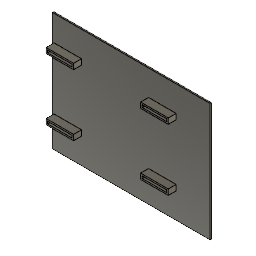
etage v3 (Autodesk Fusion 360 design; units mm, degrees)
Autodesk Fusion 360 part; units mm, degrees
sketch "Sketch1" plane through (0, 0, 0) normal (0, 1, 0) x (1, 0, 0)
  line L0 (0, 0) -> (200, 0)
  line L1 (200, 0) -> (200, -150)
  line L2 (200, -150) -> (0, -150)
  line L3 (0, -150) -> (0, 0)
  dimension "d1" = 200
  dimension "d2" = 150
extrude "Extrude1" add sketch "Sketch1" along normal blind 2
sketch "Sketch2" plane through (0, 0, 0) normal (0, -1, 0) x (1, 0, 0)
  line L0 (200, 150) -> (0, 150)
  line L1 (0, 150) -> (0, 0)
  line L2 (0, 0) -> (200, 0)
  line L3 (200, 0) -> (200, 150)
  line L4 (4, 112.5) -> (35, 112.5)
  line L5 (35, 112.5) -> (35, 115.5)
  line L6 (35, 115.5) -> (4, 115.5)
  line L7 (4, 115.5) -> (4, 112.5)
  line L8 (37, 117.5) -> (2, 117.5)
  line L9 (2, 117.5) -> (2, 110.5)
  line L10 (2, 110.5) -> (37, 110.5)
  line L11 (37, 110.5) -> (37, 117.5)
  line L12 (200, 150) -> (0, 150)
  line L13 (0, 150) -> (0, 0)
  line L14 (0, 0) -> (200, 0)
  line L15 (200, 0) -> (200, 150)
  line L16 (2, 110.5) -> (37, 110.5)
  line L17 (200, 150) -> (0, 150)
  line L18 (0, 150) -> (0, 0)
  line L19 (0, 150) -> (0, 0)
  line L20 (35, 37.5) -> (35, 34.5)
  line L21 (0, 0) -> (200, 0)
  line L22 (122, 39.5) -> (157, 39.5)
  line L23 (35, 112.5) -> (35, 115.5)
  line L24 (37, 110.5) -> (2, 110.5)
  line L25 (2, 110.5) -> (2, 117.5)
  line L26 (2, 117.5) -> (37, 117.5)
  line L27 (37, 117.5) -> (37, 110.5)
  dimension "d5" = 31
  dimension "d6" = 3
  dimension "d7" = 35
  dimension "d8" = 7
  dimension "d9" = 2
  dimension "d10" = 2
  dimension "d18" = 32.5
  dimension "d19" = 2
  measures "d5" distance of L1.end
  measures "d7" distance of L1.end
  measures "d9" distance of L6 L8
  measures "d10" distance of L5 L11
  measures "d17" distance of L16
  measures "d18" distance of L8 L17
  measures "d19" distance of L9 L18
  measures "d37" distance of L22
extrude "Extrude2" add sketch "Sketch2" along normal blind 10 contours L8 L9 L10 L11 L16 L24 L25 L26 L27
sketch "Sketch3" plane through (0, 0, 0) normal (0, -1, 0) x (1, 0, 0)
  line L0 (200, 150) -> (0, 150)
  line L1 (0, 150) -> (0, 0)
  line L2 (0, 0) -> (200, 0)
  line L3 (200, 0) -> (200, 150)
  line L4 (4, 37.5) -> (35, 37.5)
  line L5 (35, 37.5) -> (35, 34.5)
  line L6 (35, 34.5) -> (4, 34.5)
  line L7 (4, 34.5) -> (4, 37.5)
  line L8 (2, 39.5) -> (37, 39.5)
  line L9 (37, 39.5) -> (37, 32.5)
  line L10 (37, 32.5) -> (2, 32.5)
  line L11 (2, 32.5) -> (2, 39.5)
  line L12 (2, 110.5) -> (37, 110.5)
  line L13 (0, 150) -> (0, 0)
  line L14 (37, 110.5) -> (2, 110.5)
  line L15 (2, 110.5) -> (2, 117.5)
  line L16 (2, 117.5) -> (37, 117.5)
  line L17 (37, 117.5) -> (37, 110.5)
  dimension "d11" = 3
  dimension "d12" = 31
  dimension "d13" = 2
  dimension "d14" = 7
  dimension "d15" = 35
  dimension "d16" = 2
  dimension "d17" = 71
  dimension "d20" = 2
  measures "d12" distance of L1.end
  measures "d13" distance of L4 L8
  measures "d14" distance of L8 L10
  measures "d15" distance of L9 L11
  measures "d16" distance of L5 L9
  measures "d17" distance of L8 L12
  measures "d20" distance of L11 L13
extrude "Extrude3" add sketch "Sketch3" along normal blind 10 contours L8 L9 L10 L11
sketch "Sketch4" plane through (0, 0, 0) normal (0, -1, 0) x (1, 0, 0)
  line L0 (124, 37.5) -> (155, 37.5)
  line L1 (155, 37.5) -> (155, 34.5)
  line L2 (155, 34.5) -> (124, 34.5)
  line L3 (124, 34.5) -> (124, 37.5)
  line L4 (122, 39.5) -> (157, 39.5)
  line L5 (157, 39.5) -> (157, 32.5)
  line L6 (157, 32.5) -> (122, 32.5)
  line L7 (122, 32.5) -> (122, 39.5)
  line L8 (35, 37.5) -> (35, 34.5)
  line L9 (0, 0) -> (200, 0)
  dimension "d21" = 31
  dimension "d22" = 3
  dimension "d23" = 35
  dimension "d24" = 7
  dimension "d25" = 2
  dimension "d26" = 2
  dimension "d28" = 89
  dimension "d29" = 32.5
  measures "d25" distance of L3 L7
  measures "d26" distance of L2 L6
  measures "d28" distance of L3 L8
  measures "d29" distance of L6 L9
sketch "Sketch5" plane through (0, 0, 0) normal (0, -1, 0) x (1, 0, 0)
  line L0 (124, 115.5) -> (155, 115.5)
  line L1 (155, 115.5) -> (155, 112.5)
  line L2 (155, 112.5) -> (124, 112.5)
  line L3 (124, 112.5) -> (124, 115.5)
  line L4 (122, 117.5) -> (157, 117.5)
  line L5 (157, 117.5) -> (157, 110.5)
  line L6 (157, 110.5) -> (122, 110.5)
  line L7 (122, 110.5) -> (122, 117.5)
  line L8 (122, 39.5) -> (157, 39.5)
  line L9 (35, 112.5) -> (35, 115.5)
  dimension "d30" = 31
  dimension "d31" = 3
  dimension "d32" = 35
  dimension "d33" = 7
  dimension "d35" = 2
  dimension "d36" = 2
  dimension "d37" = 71
  dimension "d38" = 89
  measures "d35" distance of L3 L7
  measures "d36" distance of L2 L6
  measures "d37" distance of L6 L8
  measures "d38" distance of L3 L9
extrude "Extrude4" add sketch "Sketch4" along normal blind 10
extrude "Extrude5" add sketch "Sketch5" along normal blind 10
